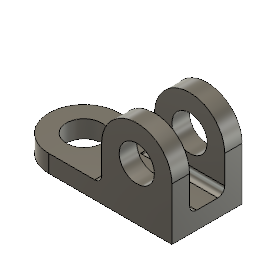
_practice4.5e542916-cbe9-4d14-8ece-5c067d7a398d (Autodesk Fusion 360 design; units mm, degrees)
Autodesk Fusion 360 part; units mm, degrees
sketch "Sketch5" plane through (0, 0, 0) normal (0, 0, 1) x (1, 0, 0)
  line L0 (0, 0) -> (114.3, 0)
  line L1 (114.3, 0) -> (114.3, 38.1)
  line L2 (114.3, 63.5) -> (104.14, 63.5)
  line L3 (0, 12.7) -> (0, 0)
  circle A0 centre (88.9, 38.1) radius 12.7
  arc A1 (114.3, 38.1) -> (63.5, 38.1) centre (88.9, 38.1) ccw
  line L4 (63.5, 38.1) -> (63.5, 12.7)
  line L5 (63.5, 12.7) -> (60.96, 12.7)
  line L6 (60.96, 12.7) -> (0, 12.7)
  dimension "d17" = 114.3
  dimension "d18" = 63.5
  dimension "d19" = 25.4
  dimension "d21" = 25.4
  dimension "d22" = 25.4
  measures "d21" diameter of A0
  measures "d22" distance of L0.start
extrude "Extrude4" add sketch "Sketch5" along normal blind 50.8
sketch "Sketch6" plane through (0, 12.7, 0) normal (0, 1, 0) x (-1, 0, 0)
  line L0 (-63.5, 0) -> (0, 0)
  line L1 (0, 0) -> (0, 50.8)
  line L2 (0, 50.8) -> (-63.5, 50.8)
  line L3 (-63.5, 50.8) -> (-63.5, 0)
  circle A0 centre (-25.4, 25.4) radius 12.7
  arc A1 (-25.4, 0) -> (-25.4, 50.8) centre (-25.4, 25.4) ccw
  dimension "d25" = 25.4
  measures "d25" diameter of A0
extrude "Extrude5" cut sketch "Sketch6" against normal blind 15.24 contours L0 L1 A1 | L1 L2 A1 | A0
sketch "Sketch7" plane through (63.5, 0, 0) normal (-1, 0, 0) x (0, 0, 1)
  line L0 (0, 38.1) -> (0, 12.7)
  line L1 (0, 12.7) -> (50.8, 12.7)
  line L2 (50.8, 12.7) -> (50.8, 38.1)
  line L3 (50.8, 38.1) -> (0, 38.1)
  line L4 (12.7, 63.5) -> (38.1, 63.5)
  line L5 (38.1, 63.5) -> (38.1, 12.7)
  line L6 (38.1, 12.7) -> (12.7, 12.7)
  line L7 (12.7, 12.7) -> (12.7, 63.5)
extrude "Extrude6" cut sketch "Sketch7" against normal blind 60.96 contours L3 L4 L5 L7 | L1 L3 L5 L6 L7
fillet "Fillet1" radius 5.08 1 edges at (63.5, 12.7, 44.45)
fillet "Fillet2" radius 5.08 1 edges at (63.5, 12.7, 6.35)
fillet "Fillet3" radius 5.08 1 edges at (86.36, 12.7, 12.7)
fillet "Fillet4" radius 5.08 1 edges at (86.36, 12.7, 38.1)
